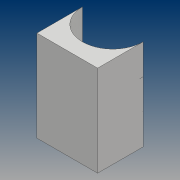
# Autodesk Inventor part: 38 (51433.628 mm^3)
Saved by Autodesk Inventor 2018 (Build 220112000, 112)
## iProperties
Created: 2020-09-18
Part Number: 38 (51433.628 mm^3)
Material: 一般
Document SubType Name: Modeling
Designer: 88697
Density: 1 g/cm^3
Appearance: 預設
Author: 88697
Autodesk Inventor part; units mm, degrees
ref_plane "YZ Plane" through (0, 0, 0) normal (1, 0, 0) x (0, 1, 0)
ref_plane "XZ Plane" through (0, 0, 0) normal (0, 1, 0) x (-1, 0, 0)
ref_plane "XY Plane" through (0, 0, 0) normal (0, 0, 1) x (1, 0, 0)
sketch "草圖1" plane through (0, 0, 0) normal (0, 0, 1) x (1, 0, 0)
  line L0 (0, 0) -> (40, 0)
  line L1 (40, 0) -> (40, 30)
  line L2 (40, 30) -> (0, 30)
  line L3 (0, 30) -> (0, 0)
  dimension "d0" = 40
  dimension "d1" = 30
  constraints: 8 end point, 2 parallel, 1 horizontal, 1 perpendicular
  measures "d0" distance of L0.start L0.end
  measures "d1" distance of L2.end L0.start
extrude "擠出1" add sketch "草圖1" along normal blind 20
sketch "草圖2" plane through (0, 0, 20) normal (0, 0, 1) x (1, 0, 0)
  line L0 (0, 30) -> (0, 0) projected
  line L1 (0, 0) -> (40, 0) projected
  line L2 (40, 30) -> (40, 0)
  line L3 (40, 0) -> (0, 0)
  line L4 (0, 0) -> (0, 30)
  line L5 (40, 30) -> (0, 30) construction
  line L6 (0, 30) -> (20, 10)
  line L7 (20, 10) -> (40, 30)
  dimension "d4" = 20
  dimension "d5" = 20
  constraints: 10 end point, 1 parallel
  measures "d4" distance from line of L0 L6.end
  measures "d5" distance from line of L5 L6.end
extrude "擠出2" add sketch "草圖2" along normal blind 20
sketch "草圖3" plane through (0, 0, 40) normal (0, 0, 1) x (1, 0, 0)
  line L0 (40, 30) -> (20, 10) construction
  arc A0 (0, 29.9839) -> (40, 30) centre (20, 30) ccw
  line L1 (0, 30) -> (0, 0) projected
  line L2 (0, 29.9839) -> (0, 0)
  line L3 (0, 0) -> (40, 0)
  line L4 (40, 0) -> (40, 30) projected
  line L5 (40, 0) -> (40, 30)
  constraints: 6 end point, 3 point on circle, 2 collinear, 1 centre point, 1 perpendicular
extrude "擠出3" add sketch "草圖3" along normal blind 20
